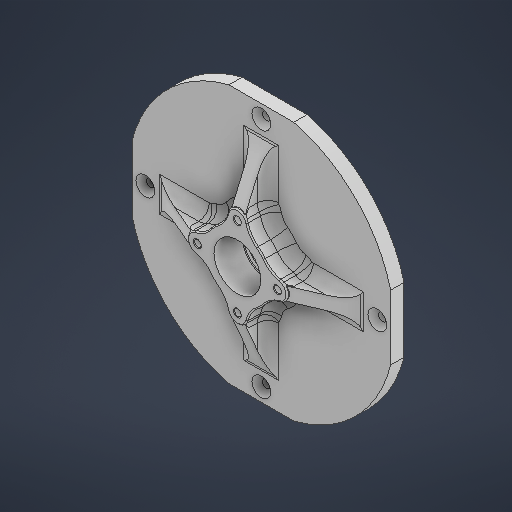
# Autodesk Inventor part: plate_lower
Saved by Autodesk Inventor 2027.1 (Build 311270010, 270A)
## iProperties
Created: 2026-10-07
Part Number: plate_lower
Material: Generisch
Document SubType Name: Modeling
Designer: luca
Density: 1 g/cm^3
Appearance: Vorgabe
Author: luca
Autodesk Inventor part; units mm, degrees
ref_plane "YZ Plane" through (0, 0, 0) normal (1, 0, 0) x (0, 1, 0)
ref_plane "XZ Plane" through (0, 0, 0) normal (0, 1, 0) x (-1, 0, 0)
ref_plane "XY Plane" through (0, 0, 0) normal (0, 0, 1) x (1, 0, 0)
sketch "Skizze1" plane through (0, 0, 0) normal (0, 1, 0) x (-1, 0, 0)
  circle A0 centre (0, 0) radius 100
  dimension "d0" = 200
  constraints: 1 centre point, 1 coincident
  measures "d0" diameter of A0
extrude "Extrusion1" add sketch "Skizze1" along normal blind 10
sketch "Skizze2" plane through (0, 10, 0) normal (0, 1, 0) x (1, 0, 0)
  circle A0 centre (0, 0) radius 100 projected
  circle A1 centre (-87, 0) radius 3.1
  dimension "d3" = 6.2
  dimension "d4" = 87
  dimension "d5" = 200
  constraints: 1 centre point, 1 horizontal alignment
  measures "d3" diameter of A1
  measures "d4" distance of A1.centre A0.centre
  measures "d5" diameter of A0
extrude "Extrusion2" cut sketch "Skizze2" against normal through all contours A1
chamfer "Fasen1" distance 4 angle 45 1 edges at (-90.1, 0, 0)
sketch "Skizze3" plane through (0, 10, 0) normal (0, 1, 0) x (1, 0, 0)
  circle A0 centre (-87, 0) radius 3.1 projected
  circle A1 centre (0, 0) radius 100 projected
  line L0 (-97, -24.3105) -> (-97, 24.3105)
  circle A2 centre (0, 0) radius 100 projected
  point P0 (-97, -24.3105)
  dimension "d11" = 10
  constraints: 2 end point, 1 point on circle, 1 vertical, 2 other
  measures "d11" distance from line of A0.centre L0
extrude "Extrusion3" cut sketch "Skizze3" against normal through all contours L0 A1 picked at (-97.7491, 4.0825)
pattern_circular "Runde Anordnung3" count 4 over 360 about axis through (0, -10, 0) along (0, 1, 0) of "Extrusion2", "Fasen1"
pattern_circular "Runde Anordnung4" count 4 over 360 about axis through (0, -10, 0) along (0, 1, 0) of "Extrusion3"
sketch "Sketch4" plane through (0, 0, 0) normal (0, -1, 0) x (1, 0, 0)
  circle A0 centre (0, 0) radius 9
  dimension "d26" = 18
  constraints: 1 centre point, 1 coincident
  measures "d26" diameter of A0
extrude "Extrusion4" cut sketch "Sketch4" against normal through all
sketch "Sketch5" plane through (0, 10, 0) normal (0, 1, 0) x (1, 0, 0)
  circle A0 centre (0, 0) radius 9 projected
  circle A1 centre (0, 0) radius 17.525
  dimension "d29" = 35.05
  constraints: 1 centre point, 1 coincident
  measures "d29" diameter of A1
extrude "Extrusion5" cut sketch "Sketch5" against normal through all
sketch "Sketch6" plane through (0, 0, 0) normal (0, -1, 0) x (1, 0, 0)
  circle A0 centre (0, 0) radius 25
  circle A1 centre (0, 0) radius 17.525 projected
  dimension "d32" = 50
  constraints: 1 centre point, 1 coincident
  measures "d32" diameter of A0
extrude "Extrusion6" add sketch "Sketch6" along normal blind 18
sketch "Sketch7" plane through (0, 10, 0) normal (0, 1, 0) x (1, 0, 0)
  circle A0 centre (0, 0) radius 17.525 projected
  circle A1 centre (0, 0) radius 15
  dimension "d35" = 30
  constraints: 1 centre point, 1 coincident
  measures "d35" diameter of A1
extrude "Extrusion7" add sketch "Sketch7" against normal blind 3
sketch "Sketch8" plane through (0, 0, 0) normal (0, -1, 0) x (1, 0, 0)
  circle A0 centre (30, 0) radius 2.55
  circle A1 centre (30, 0) radius 7.5
  circle A2 centre (0, 0) radius 25 projected
  arc A3 (31.6761, -7.3103) -> (20.081, -14.8914) centre (36.1458, -26.8045) ccw
  arc A4 (20.081, 14.8914) -> (31.6761, 7.3103) centre (36.1458, 26.8045) ccw
  dimension "d38" = 5.1
  dimension "d39" = 30
  dimension "d40" = 15
  dimension "d41" = 20
  dimension "d42" = 20
  constraints: 8 point on circle, 4 centre point, 4 tangent, 1 coincident, 1 horizontal alignment
  measures "d38" diameter of A0
  measures "d39" distance of A0.centre point (0, 0)
  measures "d40" diameter of A1
  measures "d41" radius of A3
  measures "d42" radius of A4
extrude "Extrusion8" add sketch "Sketch8" along normal up to surface (18 mm away) contours A1 A2 | A1 A2 A4 | A3 A2 A1 picked at (26.3272, 3.8714)
sketch "Sketch9" plane through (0, -18, 0) normal (0, -1, 0) x (1, 0, 0)
  circle A0 centre (30, 0) radius 2.55 projected
  point P0 (0, 0)
extrude "Extrusion9" cut sketch "Sketch9" against normal through all
pattern_circular "Circular Pattern5" count 4 over 360 about axis through (0, 10, 0) along (0, -1, 0) of "Extrusion9", "Extrusion8"
sketch "Sketch11" plane through (0, 0, 0) normal (0, 0, 1) x (1, 0, 0)
  line L0 (97, 0) -> (24.3105, 0) projected
  line L1 (37.5, -18) -> (31.6761, -18) projected
  line L2 (33.5, -18) -> (75.5, 0)
  line L3 (33.5, -18) -> (33.5, 0)
  point P0 (0, 0)
  dimension "d50" = 38
  dimension "d53" = 4
  constraints: 4 end point, 3 point on line, 1 perpendicular
  measures "d50" horizontal distance of L1.start L2.end
  measures "d53" distance of L1.start L2.start
extrude "Extrusion10" add sketch "Sketch11" along normal mid plane 10
chamfer "Chamfer2" distance 0.9 angle 45 16 edges at (37.5, -18, 0) (25.2012, -18, -10.0648) (17.6777, -18, -17.6777) (10.0648, -18, -25.2012) (0, -18, -37.5) (-10.0648, -18, -25.2012) (-17.6777, -18, -17.6777) (-25.2012, -18, -10.0648) (-37.5, -18, 0) (-25.2012, -18, 10.0648) (-17.6777, -18, 17.6777) (-10.0648, -18, 25.2012) (0, -18, 37.5) (10.0648, -18, 25.2012) (17.6777, -18, 17.6777) (25.2012, -18, 10.0648)
fillet "Fillet1" radius 10 2 edges at (35.5902, -8.55, 5) (35.5902, -8.55, -5)
pattern_circular "Circular Pattern6" count 4 over 360 about axis through (0, 10, 0) along (0, -1, 0) of "Extrusion10", "Fillet1"
fillet "Fillet2" radius 8 36 edges at (32.8045, 0, 6.9559) (36.3413, 0, 5.3638) (57.2569, 0, 5) (17.6777, 0, 17.6777) (10.0648, 0, 25.2012) (6.9559, 0, 32.8045) (5.3638, 0, 36.3413) (5, 0, 57.2569) (25.2012, 0, 10.0648) (-17.6777, 0, 17.6777) (-10.0648, 0, 25.2012) (-6.9559, 0, 32.8045) (-5.3638, 0, 36.3413) (-5, 0, 57.2569) (-32.8045, 0, 6.9559) (-36.3413, 0, 5.3638) (-57.2569, 0, 5) (-25.2012, 0, 10.0648) (-36.3413, 0, -5.3638) (-32.8045, 0, -6.9559) (-25.2012, 0, -10.0648) (-17.6777, 0, -17.6777) (-10.0648, 0, -25.2012) (-6.9559, 0, -32.8045) (-5.3638, 0, -36.3413) (-5, 0, -57.2569) (-57.2569, 0, -5) (5.3638, 0, -36.3413) (6.9559, 0, -32.8045) (10.0648, 0, -25.2012) (17.6777, 0, -17.6777) (25.2012, 0, -10.0648) (32.8045, 0, -6.9559) (36.3413, 0, -5.3638) (57.2569, 0, -5) (5, 0, -57.2569)
fillet "Fillet3" radius 4 12 edges at (9, 0, -75.5) (0, 0, -75.5) (-9, 0, -75.5) (75.5, 0, 9) (75.5, 0, 0) (75.5, 0, -9) (9, 0, 75.5) (0, 0, 75.5) (-9, 0, 75.5) (-75.5, 0, 9) (-75.5, 0, 0) (-75.5, 0, -9)
sketch "Sketch12" plane through (0, 0, 0) normal (1, 0, 0) x (0, 1, 0)
  line L0 (7, -17.525) -> (7, 17.525) projected
  line L1 (7, -17.525) -> (-18, -17.525) projected
  arc A0 (6.4, -18.125) -> (7, -17.525) centre (6.4, -17.525) ccw
  line L2 (6.4, -18.125) -> (4.4, -18.125)
  line L3 (4.4, -18.125) -> (3.1133, -17.525)
  line L4 (7, 0) -> (0, 0)
  line L5 (0, 7.1) -> (0, -7.1) projected
  dimension "d63" = 2
  dimension "d64" = 0.6
  dimension "d65" = 25
  constraints: 6 end point, 2 point on circle, 2 point on line, 1 centre point, 1 horizontal, 1 midpoint, 1 perpendicular, 1 tangent
  measures "d63" distance of L2.start L2.end
  measures "d64" distance between parallel lines of L1 L2
  measures "d65" angle of L1 L3
revolve "Revolution1" cut sketch "Sketch12" angle 360 about axis through (0, 7, 0) along (0, -1, 0)
chamfer "Chamfer3" distance 0.5 angle 45 8 edges at (0, -18, 27.45) (-27.45, -18, 0) (0, -18, -27.45) (27.45, -18, 0) (0, 10, -27.45) (-27.45, 10, 0) (0, 10, 27.45) (27.45, 10, 0)
